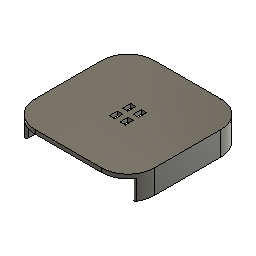
docCamera_safety (Autodesk Fusion 360 archive; units mm, degrees)
design "princeton"
Autodesk Fusion 360 part; units mm, degrees
sketch "スケッチ1" plane through (0, 0, 0) normal (0, 1, 0) x (1, 0, 0)
  line L0 (25, 45) -> (-25, 45)
  line L1 (-45, 25) -> (-45, -25)
  line L2 (-25, -45) -> (25, -45)
  line L3 (45, -25) -> (45, 25)
  line L4 (45, 45) -> (-45, -45) construction
  line L5 (-45, 45) -> (45, -45) construction
  arc A0 (-25, 45) -> (-45, 25) centre (-25, 25) ccw
  arc A1 (-45, -25) -> (-25, -45) centre (-25, -25) ccw
  arc A2 (25, -45) -> (45, -25) centre (25, -25) ccw
  arc A3 (45, 25) -> (25, 45) centre (25, 25) ccw
  dimension "d1" = 20
  constraint horizontal L0
  constraint perpendicular L0 L1
  constraint parallel L0 L2
  constraint parallel L1 L3
  constraint coincident L4 origin
  constraint coincident L5 origin
  constraint coincident L5.start L0
  constraint coincident L5.start L1
  constraint tangent L0 A0
  constraint tangent L1 A0
  constraint coincident L4.end L1
  constraint coincident L4.end L2
  constraint tangent L1 A1
  constraint tangent L2 A1
  constraint equal A0 A1
  constraint coincident L5.end L2
  constraint coincident L5.end L3
  constraint tangent L2 A2
  constraint tangent L3 A2
  constraint equal A0 A2
  constraint coincident L4.start L3
  constraint coincident L4.start L0
  constraint tangent L3 A3
  constraint tangent L0 A3
  constraint equal A0 A3
  measures "d1" radius of A0
extrude "押し出し1" add sketch "スケッチ1" along normal blind 18
sketch "スケッチ5" plane through (0, 18, 0) normal (0, 1, 0) x (-1, 0, 0)
  arc A0 (-45, -25) -> (-25, -45) centre (-25, -25) ccw
  line L0 (-25, -45) -> (25, -45)
  arc A1 (25, -45) -> (45, -25) centre (25, -25) ccw
  line L1 (45, -25) -> (45, 25)
  arc A2 (45, 25) -> (25, 45) centre (25, 25) ccw
  line L2 (25, 45) -> (-25, 45)
  arc A3 (-25, 45) -> (-45, 25) centre (-25, 25) ccw
  line L3 (-45, 25) -> (-45, -25)
  line L4 (6, -8) -> (2, -8)
  line L5 (2, -8) -> (2, -2)
  line L6 (2, -2) -> (6, -2)
  line L7 (6, -2) -> (6, -8)
  line L8 (-6, -8) -> (-6, -2)
  line L9 (-2, -2) -> (-2, -8)
  line L10 (-2, -8) -> (-6, -8)
  line L11 (-6, -2) -> (-2, -2)
  line L12 (2, 2) -> (2, 8)
  line L13 (6, 8) -> (6, 2)
  line L14 (6, 2) -> (2, 2)
  line L15 (2, 8) -> (6, 8)
  line L16 (-6, 2) -> (-6, 8)
  line L17 (-2, 8) -> (-2, 2)
  line L18 (-2, 2) -> (-6, 2)
  line L19 (-6, 8) -> (-2, 8)
  dimension "d12" = 4
  dimension "d13" = 6
  dimension "d14" = 6
  dimension "d15" = 8
  dimension "d18" = -8
  dimension "d19" = 10
  constraint horizontal L4
  constraint vertical L5
  constraint horizontal L6
  constraint vertical L7
  measures "d12" distance of L4.start L4.end
  measures "d13" distance of L4.start L6.end
  measures "d14" distance of origin L7
  measures "d15" distance of origin L4
extrude "押し出し4" cut sketch "スケッチ5" against normal blind 3 contours L4 L5 L6 L7 | L8 L9 L10 L11 | L12 L13 L14 L15 | L16 L17 L18 L19
sketch "スケッチ6" plane through (0, 0, 45) normal (0, 0, 1) x (1, 0, 0)
  line L0 (-25, 0) -> (25, 0)
  line L1 (25, 0) -> (25, 18)
  line L2 (25, 18) -> (-25, 18)
  line L3 (-25, 18) -> (-25, 0)
  line L4 (-40, 0) -> (40, 0)
  line L5 (40, 0) -> (40, 15)
  line L6 (40, 15) -> (-40, 15)
  line L7 (-40, 15) -> (-40, 0)
  dimension "d22" = 80
  dimension "d23" = 40
  dimension "d24" = 15
  constraint horizontal L4
  constraint vertical L5
  constraint horizontal L6
  constraint vertical L7
  constraint coincident origin L4
  measures "d22" distance of L4.start L4.end
  measures "d23" distance of origin L7
  measures "d24" distance of origin L6
extrude "押し出し5" cut sketch "スケッチ6" against normal through all contours L0 L1 L3 L4 L6 | L3 L4 L6 L7 | L1 L4 L5 L6
fillet "フィレット1" radius 1 4 edges at (-40, 7.5, 38.2288) (-40, 7.5, -38.2288) (40, 7.5, -38.2288) (40, 7.5, 38.2288)
sketch "スケッチ2" plane through (0, 0, 0) normal (0, 0, 1) x (1, 0, 0)
  line L0 (-10, 18) -> (10, 18)
  line L1 (10, 18) -> (10, 33)
  line L2 (-10, 33) -> (-10, 18)
  arc A0 (10, 33) -> (-10, 33) centre (0, 33) ccw
  dimension "d4" = 20
  dimension "d5" = 10
  dimension "d6" = 15
  dimension "d7" = 18
  constraint horizontal L0
  constraint vertical L1
  constraint vertical L2
  constraint horizontal L2.start A0.centre
  constraint horizontal L1.end A0.centre
  measures "d4" distance of L0.start L0.end
  measures "d5" distance of origin L1
  measures "d6" distance of L0.start L2.start
  measures "d7" distance of origin L0
extrude "押し出し2" [suppressed]
sketch "スケッチ3" plane through (0, 18, 0) normal (0, 1, 0) x (-1, 0, 0)
  line L0 (10, -10) -> (-10, -10)
  line L1 (-10, -10) -> (-10, 10)
  line L2 (-10, 10) -> (10, 10)
  line L3 (10, 10) -> (10, -10)
  arc A0 (-45, -25) -> (-25, -45) centre (-25, -25) ccw
  line L4 (-25, -45) -> (25, -45)
  arc A1 (25, -45) -> (45, -25) centre (25, -25) ccw
  line L5 (45, -25) -> (45, 25)
  arc A2 (45, 25) -> (25, 45) centre (25, 25) ccw
  line L6 (25, 45) -> (-25, 45)
  arc A3 (-25, 45) -> (-45, 25) centre (-25, 25) ccw
  line L7 (-45, 25) -> (-45, -25)
sketch "スケッチ4" plane through (0, 0, 0) normal (0, 0, 1) x (1, 0, 0)
  line L0 (0, 40) -> (-160, 40)
  line L1 (-160, 40) -> (-160, 30)
  line L2 (-160, 30) -> (0, 30)
  line L3 (0, 30) -> (0, 40)
  circle A0 centre (-160, 40) radius 10
  line L4 (-160, 50) -> (20, 50)
  line L5 (20, 50) -> (20, 40)
  line L6 (20, 40) -> (-160, 40)
  line L7 (-160, 40) -> (-160, 50)
  circle A1 centre (20, 50) radius 10
  line L8 (20, 50) -> (50, 50)
  line L9 (50, 50) -> (50, 60)
  line L10 (50, 60) -> (20, 60)
  line L11 (20, 60) -> (20, 50)
  constraint horizontal L0
  constraint vertical L1
  constraint horizontal L2
  constraint vertical L3
  constraint coincident L0.end L1.start
  constraint horizontal L4
  constraint vertical L5
  constraint horizontal L6
  constraint vertical L7
  constraint coincident A0 L4.start
  constraint coincident L4.end L5.start
  constraint coincident L5.end A1
  constraint horizontal L8
  constraint vertical L9
  constraint horizontal L10
  constraint vertical L11
extrude "押し出し3" [suppressed]

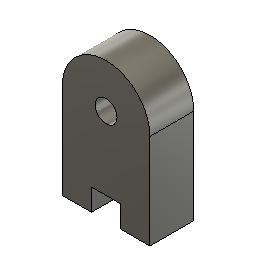
design "bottom_pin"
Autodesk Fusion 360 part; units mm, degrees
sketch "スケッチ2" plane through (0, 0, 0) normal (0, 0, 1) x (1, 0, 0)
  line L0 (-6, 3) -> (6, 3)
  line L1 (6, 3) -> (6, 13)
  line L2 (-6, 13) -> (-6, 3)
  arc A0 (6, 13) -> (-6, 13) centre (0, 13) ccw
  line L3 (-6, 3) -> (-2, 3)
  line L4 (-2, 3) -> (-2, 0)
  line L5 (-2, 0) -> (-6, 0)
  line L6 (-6, 0) -> (-6, 3)
  line L7 (6, 3) -> (2, 3)
  line L8 (2, 3) -> (2, 0)
  line L9 (2, 0) -> (6, 0)
  line L10 (6, 0) -> (6, 3)
  circle A1 centre (0, 13) radius 1.5
  dimension "d4" = 12
  dimension "d5" = 6
  dimension "d6" = 10
  dimension "d7" = 3
  dimension "d12" = 4
  dimension "d13" = 3
  constraint horizontal L0
  constraint vertical L1
  constraint vertical L2
  constraint horizontal L2.start A0.centre
  constraint horizontal L1.end A0.centre
  constraint horizontal L3
  constraint vertical L4
  constraint horizontal L5
  constraint vertical L6
  constraint horizontal L7
  constraint vertical L8
  constraint horizontal L9
  constraint vertical L10
  constraint equal L5 L9
  constraint coincident origin L5
  constraint coincident origin L9
  constraint concentric A0 A1
  measures "d4" distance of L0.start L0.end
  measures "d5" distance of origin L1
  measures "d6" distance of L0.start L2.start
  measures "d7" distance of origin L0
  measures "d12" distance of L8.end L9.end
  measures "d13" diameter of A1
extrude "押し出し2" add sketch "スケッチ2" along normal mid plane 6
sketch "スケッチ3" plane through (0, 18, 0) normal (0, 1, 0) x (-1, 0, 0)
  line L0 (10, -10) -> (-10, -10)
  line L1 (-10, -10) -> (-10, 10)
  line L2 (-10, 10) -> (10, 10)
  line L3 (10, 10) -> (10, -10)
  arc A0 (-45, -25) -> (-25, -45) centre (-25, -25) ccw
  line L4 (-25, -45) -> (25, -45)
  arc A1 (25, -45) -> (45, -25) centre (25, -25) ccw
  line L5 (45, -25) -> (45, 25)
  arc A2 (45, 25) -> (25, 45) centre (25, 25) ccw
  line L6 (25, 45) -> (-25, 45)
  arc A3 (-25, 45) -> (-45, 25) centre (-25, 25) ccw
  line L7 (-45, 25) -> (-45, -25)
sketch "スケッチ4" plane through (0, 0, 0) normal (0, 0, 1) x (1, 0, 0)
  line L0 (0, 40) -> (-160, 40)
  line L1 (-160, 40) -> (-160, 30)
  line L2 (-160, 30) -> (0, 30)
  line L3 (0, 30) -> (0, 40)
  circle A0 centre (-160, 40) radius 10
  line L4 (-160, 50) -> (20, 50)
  line L5 (20, 50) -> (20, 40)
  line L6 (20, 40) -> (-160, 40)
  line L7 (-160, 40) -> (-160, 50)
  circle A1 centre (20, 50) radius 10
  line L8 (20, 50) -> (50, 50)
  line L9 (50, 50) -> (50, 60)
  line L10 (50, 60) -> (20, 60)
  line L11 (20, 60) -> (20, 50)
  constraint horizontal L0
  constraint vertical L1
  constraint horizontal L2
  constraint vertical L3
  constraint coincident L0.end L1.start
  constraint horizontal L4
  constraint vertical L5
  constraint horizontal L6
  constraint vertical L7
  constraint coincident A0 L4.start
  constraint coincident L4.end L5.start
  constraint coincident L5.end A1
  constraint horizontal L8
  constraint vertical L9
  constraint horizontal L10
  constraint vertical L11
extrude "押し出し3" [suppressed]

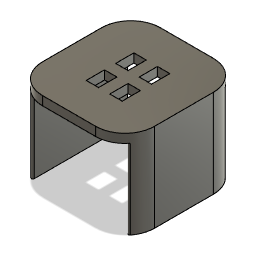
design "princeton_safety"
Autodesk Fusion 360 part; units mm, degrees
sketch "スケッチ1" plane through (0, 0, 0) normal (0, 1, 0) x (1, 0, 0)
  line L0 (9, 20) -> (-9, 20)
  line L1 (-19, 10) -> (-19, -10)
  line L2 (-9, -20) -> (9, -20)
  line L3 (19, -10) -> (19, 10)
  line L4 (19, 20) -> (-19, -20) construction
  line L5 (-19, 20) -> (19, -20) construction
  arc A0 (-9, 20) -> (-19, 10) centre (-9, 10) ccw
  arc A1 (-19, -10) -> (-9, -20) centre (-9, -10) ccw
  arc A2 (9, -20) -> (19, -10) centre (9, -10) ccw
  arc A3 (19, 10) -> (9, 20) centre (9, 10) ccw
  dimension "d1" = 10
  dimension "d28" = 40
  dimension "d29" = 38
  constraint horizontal L0
  constraint perpendicular L0 L1
  constraint parallel L0 L2
  constraint parallel L1 L3
  constraint coincident L4 origin
  constraint coincident L5 origin
  constraint coincident L5.start L0
  constraint coincident L5.start L1
  constraint tangent L0 A0
  constraint tangent L1 A0
  constraint coincident L4.end L1
  constraint coincident L4.end L2
  constraint tangent L1 A1
  constraint tangent L2 A1
  constraint equal A0 A1
  constraint coincident L5.end L2
  constraint coincident L5.end L3
  constraint tangent L2 A2
  constraint tangent L3 A2
  constraint equal A0 A2
  constraint coincident L4.start L3
  constraint coincident L4.start L0
  constraint tangent L3 A3
  constraint tangent L0 A3
  constraint equal A0 A3
  measures "d1" radius of A0
  measures "d28" distance of L0 L2
  measures "d29" distance of L1 L3
extrude "押し出し1" add sketch "スケッチ1" along normal blind 30
sketch "スケッチ5" plane through (0, 30, 0) normal (0, 1, 0) x (-1, 0, 0)
  arc A0 (-19, -10) -> (-9, -20) centre (-9, -10) ccw
  line L0 (-9, -20) -> (9, -20)
  arc A1 (9, -20) -> (19, -10) centre (9, -10) ccw
  line L1 (19, -10) -> (19, 10)
  arc A2 (19, 10) -> (9, 20) centre (9, 10) ccw
  line L2 (9, 20) -> (-9, 20)
  arc A3 (-9, 20) -> (-19, 10) centre (-9, 10) ccw
  line L3 (-19, 10) -> (-19, -10)
  line L4 (6.1, -8.1) -> (1.9, -8.1)
  line L5 (1.9, -8.1) -> (1.9, -1.9)
  line L6 (1.9, -1.9) -> (6.1, -1.9)
  line L7 (6.1, -1.9) -> (6.1, -8.1)
  line L8 (-6.1, -8.1) -> (-6.1, -1.9)
  line L9 (-1.9, -1.9) -> (-1.9, -8.1)
  line L10 (-1.9, -8.1) -> (-6.1, -8.1)
  line L11 (-6.1, -1.9) -> (-1.9, -1.9)
  line L12 (1.9, 1.9) -> (1.9, 8.1)
  line L13 (6.1, 8.1) -> (6.1, 1.9)
  line L14 (6.1, 1.9) -> (1.9, 1.9)
  line L15 (1.9, 8.1) -> (6.1, 8.1)
  line L16 (-6.1, 1.9) -> (-6.1, 8.1)
  line L17 (-1.9, 8.1) -> (-1.9, 1.9)
  line L18 (-1.9, 1.9) -> (-6.1, 1.9)
  line L19 (-6.1, 8.1) -> (-1.9, 8.1)
  dimension "d12" = 4.2
  dimension "d13" = 6.2
  dimension "d14" = 6.1
  dimension "d15" = 8.1
  dimension "d18" = -8
  dimension "d19" = 10
  constraint horizontal L4
  constraint vertical L5
  constraint horizontal L6
  constraint vertical L7
  measures "d12" distance of L4.start L4.end
  measures "d13" distance of L4.start L6.end
  measures "d14" distance of origin L7
  measures "d15" distance of origin L4
extrude "押し出し4" cut sketch "スケッチ5" against normal blind 3 contours L4 L5 L6 L7 | L8 L9 L10 L11 | L12 L13 L14 L15 | L16 L17 L18 L19
sketch "スケッチ6" plane through (0, 0, 20) normal (0, 0, 1) x (1, 0, 0)
  line L0 (-9, 0) -> (9, 0)
  line L1 (9, 0) -> (9, 30)
  line L2 (9, 30) -> (-9, 30)
  line L3 (-9, 30) -> (-9, 0)
  line L4 (-16, 0) -> (16, 0)
  line L5 (16, 0) -> (16, 27)
  line L6 (16, 27) -> (-16, 27)
  line L7 (-16, 27) -> (-16, 0)
  dimension "d22" = 32
  dimension "d23" = 16
  dimension "d24" = 27
  constraint horizontal L4
  constraint vertical L5
  constraint horizontal L6
  constraint vertical L7
  constraint coincident origin L4
  measures "d22" distance of L4.start L4.end
  measures "d23" distance of origin L7
  measures "d24" distance of origin L6
extrude "押し出し5" cut sketch "スケッチ6" against normal through all contours L0 L1 L3 L4 L6 | L3 L4 L6 L7 | L1 L4 L5 L6
fillet "フィレット1" radius 0.5 4 edges at (-16, 13.5, 17.1414) (-16, 13.5, -17.1414) (16, 13.5, -17.1414) (16, 13.5, 17.1414)
sketch "スケッチ2" plane through (0, 0, 0) normal (0, 0, 1) x (1, 0, 0)
  line L0 (-10, 18) -> (10, 18)
  line L1 (10, 18) -> (10, 33)
  line L2 (-10, 33) -> (-10, 18)
  arc A0 (10, 33) -> (-10, 33) centre (0, 33) ccw
  dimension "d4" = 20
  dimension "d5" = 10
  dimension "d6" = 15
  dimension "d7" = 18
  constraint horizontal L0
  constraint vertical L1
  constraint vertical L2
  constraint horizontal L2.start A0.centre
  constraint horizontal L1.end A0.centre
  measures "d4" distance of L0.start L0.end
  measures "d5" distance of origin L1
  measures "d6" distance of L0.start L2.start
  measures "d7" distance of origin L0
extrude "押し出し2" [suppressed]
sketch "スケッチ3" plane through (0, 18, 0) normal (0, 1, 0) x (-1, 0, 0)
  line L0 (10, -10) -> (-10, -10)
  line L1 (-10, -10) -> (-10, 10)
  line L2 (-10, 10) -> (10, 10)
  line L3 (10, 10) -> (10, -10)
  arc A0 (-45, -25) -> (-25, -45) centre (-25, -25) ccw
  line L4 (-25, -45) -> (25, -45)
  arc A1 (25, -45) -> (45, -25) centre (25, -25) ccw
  line L5 (45, -25) -> (45, 25)
  arc A2 (45, 25) -> (25, 45) centre (25, 25) ccw
  line L6 (25, 45) -> (-25, 45)
  arc A3 (-25, 45) -> (-45, 25) centre (-25, 25) ccw
  line L7 (-45, 25) -> (-45, -25)
sketch "スケッチ4" plane through (0, 0, 0) normal (0, 0, 1) x (1, 0, 0)
  line L0 (0, 40) -> (-160, 40)
  line L1 (-160, 40) -> (-160, 30)
  line L2 (-160, 30) -> (0, 30)
  line L3 (0, 30) -> (0, 40)
  circle A0 centre (-160, 40) radius 10
  line L4 (-160, 50) -> (20, 50)
  line L5 (20, 50) -> (20, 40)
  line L6 (20, 40) -> (-160, 40)
  line L7 (-160, 40) -> (-160, 50)
  circle A1 centre (20, 50) radius 10
  line L8 (20, 50) -> (50, 50)
  line L9 (50, 50) -> (50, 60)
  line L10 (50, 60) -> (20, 60)
  line L11 (20, 60) -> (20, 50)
  constraint horizontal L0
  constraint vertical L1
  constraint horizontal L2
  constraint vertical L3
  constraint coincident L0.end L1.start
  constraint horizontal L4
  constraint vertical L5
  constraint horizontal L6
  constraint vertical L7
  constraint coincident A0 L4.start
  constraint coincident L4.end L5.start
  constraint coincident L5.end A1
  constraint horizontal L8
  constraint vertical L9
  constraint horizontal L10
  constraint vertical L11
extrude "押し出し3" [suppressed]
equation "d23 = ( 32 / 2 ) * 1 mm"
